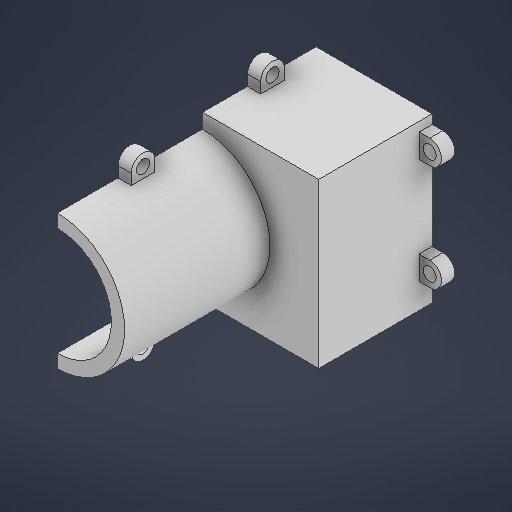
# Autodesk Inventor part: soporte p4
Saved by Autodesk Inventor 2026.1 (Build 301233020, 233B)
## iProperties
Created: 2026-01-16
Part Number: soporte p4
Material: Generic
Document SubType Name: Modeling
Designer: Marcelo
Density: 1 g/cm^3
Appearance: Default
Mass: 58.2551 g
Surface Area: 264.544 cm^2
Volume: 58.2551 cm^3
Author: Marcelo
Autodesk Inventor part; units mm, degrees
ref_plane "YZ Plane" through (0, 0, 0) normal (1, 0, 0) x (0, 1, 0)
ref_plane "XZ Plane" through (0, 0, 0) normal (0, 1, 0) x (-1, 0, 0)
ref_plane "XY Plane" through (0, 0, 0) normal (0, 0, 1) x (1, 0, 0)
sketch "Sketch1" plane through (0, 0, 0) normal (0, 0, 1) x (1, 0, 0)
  line L0 (39, -26) -> (-39, -26)
  line L1 (-39, -26) -> (-39, 26)
  line L2 (-39, 26) -> (39, 26)
  line L3 (39, 26) -> (39, -26)
  line L4 (39, -26) -> (-39, 26) construction
  line L5 (-39, -26) -> (39, 26) construction
  line L6 (44, 31) -> (-44, 31)
  line L7 (-44, 31) -> (-44, -31)
  line L8 (-44, -31) -> (44, -31)
  line L9 (44, -31) -> (44, 31)
  point P0 (0, 0)
  dimension "d0" = 78
  dimension "d1" = 52
  dimension "d2" = 5
  constraints: 20 end point, 4 parallel, 2 midpoint, 2 perpendicular, 1 horizontal, 3 other
  measures "d0" distance of L1.end L2.end
  measures "d1" distance of L0.end L1.end
  measures "d2" distance between parallel lines of L2 L6
extrude "Extrusion1" add sketch "Sketch1" along normal blind 43
sketch "Sketch2" plane through (0, 0, 43) normal (0, 0, 1) x (1, 0, 0)
  line L0 (-44, 31) -> (-44, -31) projected
  line L1 (-44, -31) -> (44, -31) projected
  line L2 (44, -31) -> (44, 31) projected
  line L3 (44, 31) -> (-44, 31) projected
  line L4 (39, -26) -> (-39, -26) projected
  line L5 (-39, -26) -> (-39, 26) projected
  line L6 (-39, 26) -> (39, 26) projected
  line L7 (39, 26) -> (39, -26) projected
  point P0 (0, 0)
extrude "Extrusion2" add sketch "Sketch2" against normal blind 5 contours L3 L2 L1 L0 | L4 L5 L6 L7
sketch "Sketch3" plane through (0, 0, 43) normal (0, 0, 1) x (1, 0, 0)
  circle A0 centre (0, 0) radius 20.5
  dimension "d7" = 41
  constraints: 1 centre point, 1 coincident
  measures "d7" diameter of A0
extrude "Extrusion3" cut sketch "Sketch3" against normal blind 5
sketch "Sketch4" plane through (0, 0, 43) normal (0, 0, 1) x (1, 0, 0)
  circle A0 centre (0, 0) radius 20.5 projected
  circle A1 centre (0, 0) radius 25.5
  dimension "d10" = 5
  constraints: 1 centre point
  measures "d10" radial gap between concentric circles of A0 A1
extrude "Extrusion4" add sketch "Sketch4" along normal blind 55
sketch "Sketch5" plane through (0, 0, 0) normal (1, 0, 0) x (0, 1, 0)
  line L0 (25.5, 43) -> (25.5, 98) projected
  line L1 (31, 0) -> (31, 43) projected
  line L2 (-31, 43) -> (31, 43) projected
  line L3 (-31, 0) -> (31, 0) projected
  line L4 (-31, 0) -> (-31, 43) projected
  line L5 (-25.5, 43) -> (-25.5, 98) projected
  line L6 (25.5, 98) -> (-25.5, 98) projected
  point P0 (0, 0)
extrude "Extrusion5" cut sketch "Sketch5" against normal blind 55
sketch "Sketch7" plane through (0, 0, 0) normal (-1, 0, 0) x (0, 0, 1)
  line L0 (0, 31) -> (43, 31) projected
  line L1 (43, 25.5) -> (98, 25.5) projected
  line L2 (70.5, 25.5) -> (70.5, 29.5)
  line L3 (21.5, 31) -> (21.5, 35)
  circle A0 centre (21.5, 35) radius 2.5
  circle A1 centre (70.5, 29.5) radius 2.5
  arc A2 (26, 35) -> (17, 35) centre (21.5, 35) ccw
  arc A3 (75, 29.5) -> (66, 29.5) centre (70.5, 29.5) ccw
  line L4 (17, 31) -> (0, 31)
  line L5 (26.9083, 31) -> (43, 31)
  line L6 (65.0917, 25.5) -> (43, 25.5)
  line L7 (75.9083, 25.5) -> (98, 25.5)
  line L8 (43, -31) -> (0, -31) projected
  line L9 (21.5, -31) -> (21.5, -35)
  line L10 (38, 26) -> (0, 26) projected
  line L11 (43, -25.5) -> (98, -25.5) projected
  line L12 (70.5, -25.5) -> (70.5, -29.5)
  circle A4 centre (70.5, -29.5) radius 2.5
  circle A5 centre (21.5, -35) radius 2.5
  arc A6 (17, -35) -> (26, -35) centre (21.5, -35) ccw
  arc A7 (66, -29.5) -> (75, -29.5) centre (70.5, -29.5) ccw
  line L13 (16.0917, -31) -> (0, -31)
  line L14 (26.9083, -31) -> (43, -31)
  line L15 (65.0917, -25.5) -> (43, -25.5)
  line L16 (75, -25.5) -> (98, -25.5)
  line L17 (17, 31) -> (17, 35)
  line L18 (26, 35) -> (26, 31)
  line L19 (66, 29.5) -> (66, 25.5)
  line L20 (75, 29.5) -> (75, 25.5)
  line L21 (17, -35) -> (17, -31)
  line L22 (26, -35) -> (26, -31)
  line L23 (66, -29.5) -> (66, -25.5)
  line L24 (75, -29.5) -> (75, -25.5)
  point P0 (0, 0)
  point P1 (19.4384, 31)
  point P2 (23.5616, 31)
  point P3 (68.4384, 25.5)
  point P4 (72.5616, 25.5)
  point P5 (23.5616, -31)
  point P6 (19.4384, -31)
  point P7 (72.5616, -25.5)
  point P8 (68.4384, -25.5)
  dimension "d40" = 4
  dimension "d41" = 4
  dimension "d42" = 5
  dimension "d43" = 5
  dimension "d44" = 2
  dimension "d45" = 2
  dimension "d47" = 4
  dimension "d48" = 4
  dimension "d49" = 5
  dimension "d50" = 5
  dimension "d51" = 2
  dimension "d52" = 2
  constraints: 40 end point, 22 point on line, 16 point on circle, 8 centre point, 8 tangent, 7 collinear, 7 vertical, 5 perpendicular, 4 coincident, 4 midpoint, 1 horizontal
  measures "d40" distance of L2.start L2.end
  measures "d41" distance of L3.start L3.end
  measures "d42" diameter of A0
  measures "d43" diameter of A1
  measures "d44" radial gap between concentric circles of A0 A2
  measures "d45" radial gap between concentric circles of A1 A3
  measures "d47" distance of L9.start L9.end
  measures "d48" distance of L12.start L12.end
  measures "d49" diameter of A4
  measures "d50" diameter of A5
  measures "d51" radial gap between concentric circles of A5 A6
  measures "d52" radial gap between concentric circles of A4 A7
extrude "Extrusion7" add sketch "Sketch7" against normal blind 5
sketch "Sketch8" plane through (0, 0, 0) normal (0, 0, -1) x (-1, 0, 0)
  line L0 (-44, 23) -> (-48, 23)
  line L1 (-44, 23) -> (-40, 23) construction
  line L2 (-44, -17) -> (-48, -17)
  line L3 (-44, 31) -> (0, 31) projected
  circle A0 centre (-48, 23) radius 2.5
  circle A1 centre (-48, -17) radius 2.5
  line L4 (-44, 28.4083) -> (-44, 31)
  line L5 (-44, -31) -> (-44, 31) projected
  arc A2 (-48, 27.5) -> (-48, 18.5) centre (-48, 23) ccw
  arc A3 (-48, -12.5) -> (-48, -21.5) centre (-48, -17) ccw
  line L6 (-44, -31) -> (-44, -23.1847)
  line L7 (-44, -10.8153) -> (-44, 16.8153)
  line L8 (-44, 29.1847) -> (-44, 31)
  line L9 (-48, 27.5) -> (-44, 27.5)
  line L10 (-48, 18.5) -> (-44, 18.5)
  line L11 (-48, -12.5) -> (-44, -12.5)
  line L12 (-48, -21.5) -> (-44, -21.5)
  point P0 (0, 0)
  point P1 (-44, 20.9384)
  point P2 (-44, 25.0616)
  point P3 (-44, -19.0616)
  point P4 (-44, -14.9384)
  dimension "d56" = 4
  dimension "d57" = 180
  dimension "d58" = 40
  dimension "d59" = 8
  dimension "d60" = 5
  dimension "d61" = 5
  dimension "d65" = 4
  dimension "d68" = 2
  dimension "d69" = 2
  constraints: 23 end point, 9 point on circle, 5 horizontal, 5 point on line, 4 centre point, 4 tangent, 2 coincident, 2 vertical, 1 collinear, 11 other
  measures "d56" distance of L0.start L0.end
  measures "d57" angle of L0 L1
  measures "d58" distance between parallel lines of L2 L0
  measures "d59" distance between parallel lines of L3 L0
  measures "d60" diameter of A0
  measures "d61" diameter of A1
  measures "d65" distance of L2.start L2.end
  measures "d68" radial gap between concentric circles of A0 A2
  measures "d69" radial gap between concentric circles of A1 A3
extrude "Extrusion8" add sketch "Sketch8" against normal blind 5
body "Solid1"
